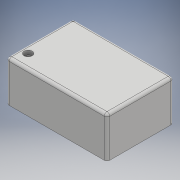
# Autodesk Inventor part: Extrusion
Saved by Autodesk Inventor 2018 (Build 220112000, 112)
## iProperties
Created: 2018-04-09
Part Number: Extrusion
Material: Generic
Document SubType Name: Modeling
Designer: anshs
Density: 1 g/cm^3
Appearance: Default
Mass: 23.3364 g
Surface Area: 205.221 cm^2
Volume: 23.3364 cm^3
Author: anshs
Autodesk Inventor part; units mm, degrees
ref_plane "YZ Plane" through (0, 0, 0) normal (1, 0, 0) x (0, 1, 0)
ref_plane "XZ Plane" through (0, 0, 0) normal (0, 1, 0) x (-1, 0, 0)
ref_plane "XY Plane" through (0, 0, 0) normal (0, 0, 1) x (1, 0, 0)
sketch "Sketch1" plane through (0, 0, 0) normal (0, 0, 1) x (1, 0, 0)
  line L0 (-15, 57.0488) -> (55, 57.0488)
  line L1 (-15, 12.0488) -> (-15, 57.0488)
  line L2 (55, 12.0488) -> (-15, 12.0488)
  line L3 (55, 57.0488) -> (55, 12.0488)
  line L4 (-17, 59.0488) -> (57, 59.0488)
  line L5 (57, 59.0488) -> (57, 10.0488)
  line L6 (57, 10.0488) -> (-17, 10.0488)
  line L7 (-17, 10.0488) -> (-17, 59.0488)
  point P0 (0, 0)
  dimension "d0" = 74
  dimension "d1" = 49
  dimension "d2" = 2
  dimension "d3" = 2
  constraints: 16 end point, 2 parallel, 1 horizontal, 1 perpendicular
  measures "d0" distance of L4.start L4.end
  measures "d1" distance of L6.end L4.start
  measures "d2" distance between parallel lines of L7 L1
  measures "d3" distance between parallel lines of L4 L0
extrude "Extrusion1" add sketch "Sketch1" along normal blind 27
sketch "Sketch2" plane through (0, 0, 27) normal (0, 0, 1) x (1, 0, 0)
  line L0 (57, 59.0488) -> (-17, 59.0488) projected
  line L1 (-17, 59.0488) -> (57, 59.0488)
  line L2 (57, 59.0488) -> (57, 10.0488)
  line L3 (57, 10.0488) -> (-17, 10.0488)
  line L4 (-17, 10.0488) -> (-17, 59.0488)
  point P0 (0, 0)
  constraints: 8 end point, 2 parallel, 1 horizontal, 1 perpendicular
extrude "Extrusion2" add sketch "Sketch2" along normal blind 3
sketch "Sketch3" plane through (0, 0, 30) normal (0, 0, 1) x (1, 0, 0)
  circle A0 centre (-11, 20.0488) radius 3
  line L0 (-17, 10.0488) -> (57, 10.0488) projected
  line L1 (-17, 59.0488) -> (-17, 10.0488) projected
  point P0 (0, 0)
  dimension "d8" = 6
  dimension "d9" = 10
  dimension "d10" = 6
  constraints: 1 centre point
  measures "d8" diameter of A0
  measures "d9" distance from line of L0 A0.centre
  measures "d10" distance from line of L1 A0.centre
extrude "Extrusion3" cut sketch "Sketch3" against normal up to next
fillet "Fillet1" radius 2 8 edges at (57, 34.5488, 30) (20, 59.0488, 30) (57, 59.0488, 15) (57, 10.0488, 15) (-17, 59.0488, 15) (-17, 34.5488, 30) (-17, 10.0488, 15) (20, 10.0488, 30)
body "Solid1"
